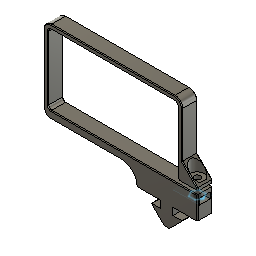
PSU-clamp v5 (Autodesk Fusion 360 design; units mm, degrees)
Autodesk Fusion 360 part; units mm, degrees
note: some values were not read from the file. Chosen so that the rebuilt part matches the saved one: which face or edge a step refers to.
sketch "Sketch1" plane through (0, 0, 0) normal (0, 0, 1) x (1, 0, 0)
  line L0 (20, 17.5) -> (0, 17.5) construction
  line L1 (0, 17.5) -> (0, 4) construction
  line L2 (20, 2.8) -> (14, 2.8)
  line L3 (14, 2.8) -> (14, 17.5)
  line L4 (6, 17.5) -> (14, 17.5)
  line L5 (11.6519, -5.8) -> (20, 2.5481)
  line L6 (6, 2.8) -> (6, 17.5) construction
  line L7 (8.3481, -5.8) -> (11.6519, -5.8)
  line L8 (6, 17.5) -> (6, 2.8)
  line L9 (0, 2.8) -> (0, 2.5481)
  line L10 (0, 2.5481) -> (8.3481, -5.8)
  line L11 (6, 2.8) -> (0, 2.8)
  line L12 (20, 2.5481) -> (20, 2.8)
  line L13 (30, 17.5) -> (-70, 17.5)
  line L14 (-66, 22.5) -> (30, 22.5)
  line L15 (30, 22.5) -> (30, 17.5)
  line L16 (20, 24.5) -> (19, 24.5)
  line L17 (17, 26.5) -> (17, 66.5)
  line L18 (20, 66.5) -> (20, 26.5)
  line L19 (-70, 17.5) -> (-71, 17.5)
  line L20 (-71, 17.5) -> (-71, 66.5)
  line L21 (-68, 66.5) -> (-68, 24.5)
  line L22 (-66, 68.5) -> (15, 68.5)
  line L23 (15, 71.5) -> (-66, 71.5)
  line L24 (20, 24.5) -> (30, 24.5)
  line L25 (30, 24.5) -> (30, 26.5)
  line L26 (30, 26.5) -> (20, 26.5)
  arc A0 (-66, 68.5) -> (-68, 66.5) centre (-66, 66.5) ccw
  arc A1 (17, 66.5) -> (15, 68.5) centre (15, 66.5) ccw
  arc A2 (-68, 24.5) -> (-66, 22.5) centre (-66, 24.5) ccw
  arc A3 (17, 26.5) -> (19, 24.5) centre (19, 26.5) ccw
  arc A4 (-66, 71.5) -> (-71, 66.5) centre (-66, 66.5) ccw
  arc A5 (20, 66.5) -> (15, 71.5) centre (15, 66.5) ccw
  line L27 (30, 17.5) -> (30, 7.5)
  line L28 (30, 7.5) -> (-10, 7.5)
  line L29 (-10, 7.5) -> (-10, 17.5)
  point P0 (0, 4)
  point P1 (17, 24.5)
  dimension "d2" = 13.5
  dimension "d3" = 8
  dimension "d5" = 6
  dimension "d10" = 14
  dimension "d12" = 5
  dimension "d13" = 3
  dimension "d16" = 30
  dimension "d22" = 10
  dimension "d23" = 2
  dimension "d28" = 85
  dimension "d29" = 46
  dimension "d30" = 3
  dimension "d31" = 3
  dimension "d32" = 2
  dimension "d36" = 30
  dimension "d40" = 2
  dimension "d55" = 20
  dimension "d56" = 3.3038
  dimension "d57" = 11.806
  dimension "d58" = 6
  dimension "d59" = 8.6
  dimension "d60" = 14.7
  dimension "d62" = 10
  dimension "d63" = 40
  constraint horizontal L0
  constraint vertical L1
  constraint coincident P0 L1.end
  constraint vertical L6
  constraint coincident L4.start L0
  constraint coincident L9.start L1
  constraint coincident L9.end L1
  constraint horizontal L13
  constraint horizontal L14
  constraint vertical L15
  constraint coincident L0 L13.start
  constraint horizontal L16
  constraint vertical L17
  constraint vertical L18
  constraint horizontal L19
  constraint vertical L20
  constraint vertical L21
  constraint horizontal L22
  constraint horizontal L23
  constraint horizontal L24
  constraint vertical L25
  constraint horizontal L26
  constraint tangent L21 A0
  constraint tangent L22 A0
  constraint tangent L22 A1
  constraint tangent L17 A1
  constraint equal A0 A1
  constraint tangent L14 A2
  constraint tangent L21 A2
  constraint equal A0 A2
  constraint coincident P1 L16
  constraint coincident P1 L17
  constraint tangent L16 A3
  constraint tangent L17 A3
  constraint equal A0 A3
  constraint concentric A0 A4
  constraint tangent L23 A4
  constraint concentric A1 A5
  constraint tangent L23 A5
  constraint perpendicular L13 L27
  constraint perpendicular L27 L28
  constraint coincident L13 L29.end
  constraint perpendicular L13 L29
  measures "d2" distance of L0.end P0
  measures "d3" distance of L4.start L3.end
  measures "d5" distance of L1 L6
  measures "d10" distance of origin L3
  measures "d12" distance of L13.start L14.end
  measures "d13" distance of L16.start P1
  measures "d16" distance of P0 L15
  measures "d22" distance of L16.start L24.end
  measures "d23" distance of L16.start L18.end
  measures "d28" distance of L17 L21
  measures "d29" distance of L14 L22
  measures "d30" distance of L20 L21
  measures "d31" distance of L22 L23
  measures "d32" radius of A0
  measures "d36" horizontal distance of P0 L24.end
  measures "d40" distance of L14 L24
  measures "d55" distance of L9.start L2.start
  measures "d56" distance of L5.start L7.start
  measures "d57" distance of L5.start L5.end
  measures "d58" distance of L2.end L2.start
  measures "d59" vertical distance of L2.end L5.start
  measures "d60" distance of L6.start L4.start
  measures "d62" distance of L13.start L27.end
  measures "d63" distance of L27.end L28.end
extrude "Extrude1" add sketch "Sketch1" along normal blind 10
fillet "Fillet3" radius 5 1 edges at (-71, 17.5, 5)
chamfer "Chamfer1" distance 10 angle 45 1 edges at (20, 26.5, 5)
sketch "Sketch2" plane through (0, 22.5, 0) normal (0, 1, 0) x (-1, 0, 0)
  line L0 (-30, 0) -> (66, 0)
  line L1 (66, 0) -> (66, 10)
  line L2 (66, 10) -> (-30, 10)
  line L3 (-30, 10) -> (-30, 0)
  circle A0 centre (-25, 5) radius 4.5
  circle A1 centre (-25, 5) radius 2
  dimension "d38" = 9
  dimension "d39" = 4
  constraint concentric A0 A1
  measures "d38" diameter of A0
  measures "d39" diameter of A1
extrude "Extrude2" cut sketch "Sketch2" along normal blind 20 and the other way blind 20 contours A1
extrude "Extrude3" cut sketch "Sketch2" along normal blind 10 from surface at 5 contours A0
sketch "Sketch3" plane through (0, 17.5, 0) normal (0, -1, 0) x (1, 0, 0)
  circle A0 centre (25, 5) radius 2
  line L0 (14, 0) -> (30, 0)
  line L1 (30, 0) -> (30, 10)
  line L2 (30, 10) -> (14, 10)
  line L3 (14, 10) -> (14, 0)
  line L4 (29.0414, 5.0056) -> (27.0159, 8.5028)
  line L5 (27.0159, 8.5028) -> (22.9744, 8.4972)
  line L6 (22.9744, 8.4972) -> (20.9586, 4.9944)
  line L7 (20.9586, 4.9944) -> (22.9841, 1.4972)
  line L8 (22.9841, 1.4972) -> (27.0256, 1.5028)
  line L9 (27.0256, 1.5028) -> (29.0414, 5.0056)
  point P0 (25, 5)
  dimension "d48" = 3.5
  constraint coincident P0 A0.centre
  measures "d48" distance of P0 L9
extrude "Extrude4" cut sketch "Sketch3" along normal blind -2.5 and the other way blind 2 contours L4 L5 L6 L7 L8 L9
fillet "Fillet4" radius 10 1 edges at (-10, 17.5, 5)
chamfer "Chamfer2" distance 0.5 angle 45 44 edges at (-42.999, 17.5, 0) (-12.9283, 14.5717, 0) (-69.5356, 18.9645, 0) (-10, 7.501, 0) (-71, 44.5, 0) (-69.5355, 70.0355, 0) (-25.5, 71.5, 0) (18.5355, 70.0355, 0) (20, 51.499, 0) (24.999, 31.499, 0) (29.999, 26.5, 0) (30, 25.5, 0) (24.5, 24.5, 0) (17.5858, 25.0858, 0) (17, 46.5, 0) (16.4142, 67.9142, 0) (30, 15, 0) (-25.5, 68.5, 0) (-18, 22.5, 0) (-67.4142, 67.9142, 0) (-67.4142, 23.0858, 0) (-68, 45.5, 0) (-42.999, 17.5, 10) (-12.9283, 14.5717, 10) (-69.5356, 18.9645, 10) (-10, 7.501, 10) (-71, 44.5, 10) (-69.5355, 70.0355, 10) (-25.5, 71.5, 10) (18.5355, 70.0355, 10) (20, 51.499, 10) (24.999, 31.499, 10) (29.999, 26.5, 10) (30, 25.5, 10) (24.5, 24.5, 10) (17.5858, 25.0858, 10) (17, 46.5, 10) (16.4142, 67.9142, 10) (30, 15, 10) (-25.5, 68.5, 10) (-18, 22.5, 10) (-67.4142, 67.9142, 10) (-67.4142, 23.0858, 10) (-68, 45.5, 10)
sketch "Sketch4" plane through (30, 0, 0) normal (1, 0, 0) x (0, 0, -1)
  line L0 (-9.5, 22.5) -> (-9.5, 7.5)
  line L1 (-9.5, 7.5) -> (-0.5, 7.5)
  line L2 (-0.5, 7.5) -> (-0.5, 22.5)
  line L3 (-0.5, 22.5) -> (-9.5, 22.5)
  line L4 (-1.5, 16) -> (-8.5, 16)
  line L5 (-8.5, 16) -> (-8.5, 20)
  line L6 (-8.5, 20) -> (-1.5, 20)
  line L7 (-1.5, 20) -> (-1.5, 16)
  line L8 (-1.5, 16) -> (-8.5, 20) construction
  line L9 (-8.5, 16) -> (-1.5, 20) construction
  line L10 (0, 17.5) -> (-10, 17.5)
  dimension "d68" = 7
  dimension "d69" = 4
  dimension "d70" = 2.5
  constraint horizontal L4
  constraint perpendicular L4 L5
  constraint parallel L4 L6
  constraint parallel L5 L7
  measures "d68" distance of L5.end L6.end
  measures "d69" distance of L4.end L5.end
  measures "d70" distance of L3 L6
extrude "Extrude5" cut sketch "Sketch4" against normal blind 5 contours L4 L5 L7 L10 | L5 L6 L7 L10
extrude "Extrude6" cut sketch "Sketch3" along normal blind 1.5 and the other way blind 2.5 contours L4 L5 L6 L7 L8 L9
equation "d1 = 20 mm"
equation "d5 = ( d1 - d3 ) / 2"
equation "d13 = d30"
equation "d31 = d30"
equation "d36 = d16"
equation "d60 = 4.70 mm + 10 mm"
